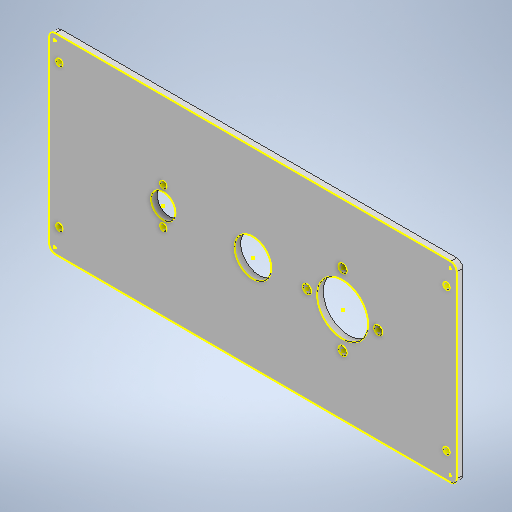
# Autodesk Inventor part: canon_plate_motor
Saved by Autodesk Inventor 2025.1 (Build 291241000, 241)
## iProperties
Created: 2024-10-05
Part Number: canon_plate_motor
Material: 一般
Document SubType Name: Modeling
Designer: yuki0520
Density: 1 g/cm^3
Appearance: 既定
Author: yuki0520
Autodesk Inventor part; units mm, degrees
ref_plane "YZ Plane" through (0, 0, 0) normal (1, 0, 0) x (0, 1, 0)
ref_plane "XZ Plane" through (0, 0, 0) normal (0, 1, 0) x (-1, 0, 0)
ref_plane "XY Plane" through (0, 0, 0) normal (0, 0, 1) x (1, 0, 0)
sketch "スケッチ1" plane through (0, 0, 0) normal (0, 0, 1) x (1, 0, 0)
  circle A0 centre (0, 0) radius 77
  circle A1 centre (0, 0) radius 9
  circle A2 centre (44, 0) radius 12.5
  circle A3 centre (-44, 0) radius 6
  line L0 (100, -77) -> (-100, -77)
  line L1 (-100, -77) -> (-100, 77)
  line L2 (-100, 77) -> (100, 77)
  line L3 (100, 77) -> (100, -77)
  line L4 (100, -77) -> (-100, 77) construction
  line L5 (-100, -77) -> (100, 77) construction
  line L6 (-100, 0) -> (100, 0)
  line L7 (-100, 47) -> (100, 47)
  circle A4 centre (-95, 35.5) radius 1.6
  circle A5 centre (-95, -34.5) radius 1.6
  circle A6 centre (95, 35.5) radius 1.6
  circle A7 centre (95, -34.5) radius 1.6
  circle A8 centre (-44, 0) radius 9
  circle A9 centre (44, 0) radius 17.5
  circle A10 centre (-44, 9) radius 1.6
  circle A11 centre (-44, -9) radius 1.6
  circle A12 centre (44, 17.5) radius 2.05
  circle A13 centre (26.5, 0) radius 2.05
  circle A14 centre (44, -17.5) radius 2.05
  circle A15 centre (61.5, 0) radius 2.05
  line L8 (-100, -47) -> (100, -47)
  dimension "d20" = 18
  dimension "d21" = 35
  dimension "d0" = 154
  dimension "d1" = 18
  dimension "d2" = 25
  dimension "d3" = 12
  dimension "d4" = 44
  dimension "d5" = 44
  dimension "d6" = 200
  dimension "d7" = 30
  dimension "d8" = 3.2
  dimension "d9" = 3.2
  dimension "d10" = 3.2
  dimension "d11" = 3.2
  dimension "d12" = 5
  dimension "d15" = 5
  dimension "d16" = 5
  dimension "d17" = 70
  dimension "d18" = 5
  dimension "d19" = 70
  dimension "d22" = 3.2
  dimension "d25" = 360
  dimension "d27" = 9
  dimension "d28" = 4.1
  dimension "d29" = 17.5
  dimension "d32" = 360
  dimension "d36" = 11.5
  dimension "d37" = 11.5
  dimension "d38" = 30
  constraints: 18 end point, 14 centre point, 6 point on line, 4 coincident, 4 midpoint, 3 perpendicular, 2 parallel, 2 vertical alignment, 1 horizontal, 1 tangent, 18 other
  measures "d0" diameter of A0
  measures "d1" diameter of A1
  measures "d2" diameter of A2
  measures "d3" diameter of A3
  measures "d4" distance of A2.centre A1.centre
  measures "d5" distance of A3.centre A1.centre
  measures "d6" distance of L1.end L2.end
  measures "d7" distance between parallel lines of L2 L7
  measures "d8" diameter of A4
  measures "d9" diameter of A5
  measures "d10" diameter of A6
  measures "d11" diameter of A7
  measures "d12" distance from line of L1 A5.centre
  measures "d15" distance from line of L3 A7.centre
  measures "d16" distance from line of L3 A6.centre
  measures "d17" distance of A7.centre A6.centre
  measures "d18" distance from line of L1 A4.centre
  measures "d19" distance of A5.centre A4.centre
  measures "d22" diameter of A10
  measures "d27" distance from line of L6 A10.centre
  measures "d28" diameter of A12
  measures "d29" distance from line of L6 A12.centre
  measures "d36" distance from line of L7 A4.centre
  measures "d37" distance from line of L7 A6.centre
  measures "d38" distance between parallel lines of L0 L8
extrude "押し出し1" add sketch "スケッチ1" along normal blind 3 contours L6 A15 A9 A12 A13 A1 A8 A10 A0 L7 | L6 L3 L8 A0 | A0 L8 L6 A8 A11 A1 A13 A9 A14 A15 | A0 L7 L3 L6 | A0 L6 L1 L7 | L8 L1 L6 A0 | A15 L6 A2 A13 A9 A12 | A9 A14 A13 L6 A2 A15 | A8 A10 L6 A3 | L6 A3 A8 A11
fillet "フィレット1" radius 3 4 edges at (100, 47, 1.5) (100, -47, 1.5) (-100, -47, 1.5) (-100, 47, 1.5)
sketch "スケッチ2" plane through (0, 0, 3) normal (0, 0, 1) x (1, 0, 0)
  arc A0 (-97, 47) -> (-100, 44) centre (-97, 44) ccw projected
  line L0 (-100, 44) -> (-100, -44) projected
  arc A1 (-100, -44) -> (-97, -47) centre (-97, -44) ccw projected
  line L1 (-97, -47) -> (97, -47) projected
  arc A2 (97, -47) -> (100, -44) centre (97, -44) ccw projected
  line L2 (100, -44) -> (100, 44) projected
  arc A3 (100, 44) -> (97, 47) centre (97, 44) ccw projected
  line L3 (97, 47) -> (-97, 47) projected
  circle A4 centre (-95, 35.5) radius 1.6 projected
  circle A5 centre (95, 35.5) radius 1.6 projected
  circle A6 centre (-44, 9) radius 1.6 projected
  circle A7 centre (44, 17.5) radius 2.05 projected
  circle A8 centre (61.5, 0) radius 2.05 projected
  circle A9 centre (26.5, 0) radius 2.05 projected
  circle A10 centre (-95, -34.5) radius 1.6 projected
  circle A11 centre (-44, 0) radius 6 projected
  circle A12 centre (-44, -9) radius 1.6 projected
  circle A13 centre (0, 0) radius 9 projected
  circle A14 centre (44, 0) radius 12.5 projected
  circle A15 centre (95, -34.5) radius 1.6 projected
  circle A16 centre (44, -17.5) radius 2.05 projected
equation "\"d5\" = d4"
equation "\"d17\" = d19"
equation "\"d29\" = 0.5 * d21"
equation "\"d37\" = d36"
equation "\"d38\" = d7"
